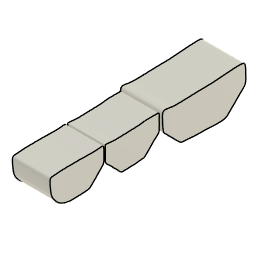
biomechanical finger (Autodesk Fusion 360 design; units mm, degrees)
Autodesk Fusion 360 part; units mm, degrees
sketch "Sketch1" plane through (0, 0, 0) normal (1, 0, 0) x (0, 1, 0)
  line L0 (-19, 9) -> (19, 9)
  line L1 (19, 9) -> (19, -9)
  line L2 (19, -9) -> (-19, -9)
  line L3 (-19, -9) -> (-19, 9)
  line L4 (-19, 9) -> (19, -9) construction
  line L5 (19, 9) -> (-19, -9) construction
  line L6 (-19, 0) -> (-44, 0) construction
  line L7 (-44, 0) -> (-69, 0) construction
  line L8 (-44, 0) -> (-44, 7.5)
  line L9 (-44, 7.5) -> (-19, 7.5)
  line L10 (-44, -7.5) -> (-19, -7.5)
  line L11 (-44, 0) -> (-44, -7.5)
  line L12 (-69, 0) -> (-69, 7.5)
  line L13 (-69, 7.5) -> (-44, 7.5)
  line L14 (-69, -7.5) -> (-44, -7.5)
  line L15 (-69, 0) -> (-69, -7.5)
  dimension "d1" = 38
  dimension "d2" = 18
  dimension "d3" = 25
  dimension "d4" = 25
  dimension "d5" = 7.5
  constraint horizontal L0
  constraint perpendicular L0 L1
  constraint parallel L0 L2
  constraint parallel L1 L3
  constraint coincident L4 origin
  constraint coincident L5 origin
  constraint midpoint L3 L6.start
  constraint perpendicular L3 L6
  constraint parallel L6 L7
  constraint perpendicular L7 L8
  constraint coincident L3 L9.end
  constraint perpendicular L3 L9
  constraint symmetric L7.start L6 L8.start
  constraint symmetric L6 L8.end L10.start
  constraint symmetric L6 L9.end L10.end
  constraint perpendicular L9 L12
  constraint perpendicular L8 L13
  constraint symmetric L12.start L7 L15.start
  constraint symmetric L7 L8.end L10.start
  constraint symmetric L7 L12.end L14.start
  measures "d1" distance of L0.start L0.end
  measures "d2" distance of L0.end L1.end
  measures "d3" distance of L6.start L6.end
  measures "d4" distance of L6.end L7.end
  measures "d5" distance of L6.end L8.end
sketch "Sketch2" plane through (0, 0, 0) normal (1, 0, 0) x (0, 1, 0)
  spline S0 degree 5 poles (26, 7) (25.7359, 7.0846) (25.2232, 7.2494) (24.5006, 7.4834) (23.6297, 7.7689) (22.6905, 8.0818) (21.884, 8.3509) (21.1781, 8.577) (20.5163, 8.7611) (19.8228, 8.9049) (19.0268, 9.0102) (18.0817, 9.0787) (16.9866, 9.1116) (15.7716, 9.1104) (14.4837, 9.0774) (13.1721, 9.0158) (11.8746, 8.9309) (10.602, 8.8299) (9.343, 8.7215) (8.0735, 8.6147) (6.764, 8.517) (5.3873, 8.4337) (3.9268, 8.3666) (2.3835, 8.3129) (0.7706, 8.267) (-0.8891, 8.2223) (-2.5676, 8.1727) (-4.2351, 8.1144) (-5.8638, 8.047) (-7.4316, 7.9759) (-8.9255, 7.9128) (-10.3394, 7.8724) (-11.6729, 7.8682) (-12.9294, 7.91) (-14.1153, 7.9996) (-15.2374, 8.1277) (-16.3028, 8.2707) (-17.3181, 8.3986) (-18.2905, 8.4817) (-19.228, 8.4975) (-20.1395, 8.4391) (-21.0354, 8.3162) (-21.9286, 8.1476) (-22.8349, 7.9564) (-23.7743, 7.7623) (-24.7697, 7.5788) (-25.8432, 7.4148) (-27.0111, 7.2746) (-28.2811, 7.159) (-29.6469, 7.0661) (-31.0894, 6.9921) (-32.5801, 6.9328) (-34.0848, 6.8844) (-35.5662, 6.8451) (-36.9876, 6.8158) (-38.3159, 6.802) (-39.5247, 6.8127) (-40.5987, 6.856) (-41.5367, 6.9349) (-42.3554, 7.0434) (-43.0947, 7.1607) (-43.8126, 7.254) (-44.5637, 7.2937) (-45.381, 7.2652) (-46.2562, 7.183) (-47.159, 7.0784) (-48.0575, 6.9862) (-48.9377, 6.9326) (-49.8227, 6.9228) (-50.7556, 6.9481) (-51.7839, 6.9924) (-52.9443, 7.038) (-54.2456, 7.0728) (-55.6718, 7.0903) (-57.1903, 7.0877) (-58.7578, 7.0655) (-60.3275, 7.0258) (-61.855, 6.9716) (-63.3064, 6.9054) (-64.6596, 6.8287) (-65.9014, 6.7425) (-66.8004, 6.6663) (-67.4206, 6.6051) (-67.8101, 6.5626) (-67.9988, 6.5409) knots 0 0 0 0 0 0 0.0125 0.025 0.0375 0.05 0.0625 0.075 0.0875 0.1 0.1125 0.125 0.1375 0.15 0.1625 0.175 0.1875 0.2 0.2125 0.225 0.2375 0.25 0.2625 0.275 0.2875 0.3 0.3125 0.325 0.3375 0.35 0.3625 0.375 0.3875 0.4 0.4125 0.425 0.4375 0.45 0.4625 0.475 0.4875 0.5 0.5125 0.525 0.5375 0.55 0.5625 0.575 0.5875 0.6 0.6125 0.625 0.6375 0.65 0.6625 0.675 0.6875 0.7 0.7125 0.725 0.7375 0.75 0.7625 0.775 0.7875 0.8 0.8125 0.825 0.8375 0.85 0.8625 0.875 0.8875 0.9 0.9125 0.925 0.9375 0.95 0.9625 0.975 0.9875 1 1 1 1 1 1
  spline S1 degree 5 poles (24.5129, -11.4787) (24.1663, -11.4324) (23.4806, -11.3421) (22.4736, -11.2136) (21.1745, -11.0562) (19.6223, -10.8825) (18.14, -10.7313) (16.7236, -10.6017) (15.3664, -10.492) (14.0584, -10.3994) (12.7852, -10.3205) (11.5285, -10.2504) (10.2679, -10.1839) (8.9836, -10.1157) (7.6581, -10.0412) (6.2784, -9.9568) (4.8385, -9.8605) (3.3396, -9.752) (1.7887, -9.6322) (0.1966, -9.5021) (-1.4231, -9.3632) (-3.0551, -9.2161) (-4.6844, -9.0606) (-6.2975, -8.8946) (-7.8824, -8.715) (-9.4273, -8.5182) (-10.9199, -8.3017) (-12.3462, -8.0641) (-13.6899, -7.807) (-14.9313, -7.5353) (-16.0458, -7.2582) (-17.0119, -6.9883) (-17.8199, -6.74) (-18.4796, -6.5277) (-19.0306, -6.365) (-19.544, -6.2627) (-20.1061, -6.2277) (-20.8056, -6.2621) (-21.7226, -6.3619) (-22.9187, -6.5182) (-24.4273, -6.7167) (-26.2439, -6.9382) (-28.3153, -7.1582) (-30.5528, -7.3503) (-32.846, -7.4887) (-35.0769, -7.551) (-37.1338, -7.5214) (-38.9249, -7.3935) (-40.3925, -7.1729) (-41.5257, -6.8802) (-42.3788, -6.555) (-43.0656, -6.2525) (-43.7166, -6.0257) (-44.4493, -5.9137) (-45.3253, -5.9238) (-46.3498, -6.0337) (-47.4939, -6.2059) (-48.71, -6.3983) (-49.9501, -6.5762) (-51.1823, -6.723) (-52.3873, -6.8359) (-53.5553, -6.9202) (-54.6829, -6.9853) (-55.7698, -7.0398) (-56.8154, -7.0861) (-57.8192, -7.1196) (-58.7823, -7.1298) (-59.7095, -7.1007) (-60.6106, -7.0114) (-61.5014, -6.8372) (-62.3961, -6.5559) (-63.3012, -6.153) (-64.2093, -5.6276) (-65.0915, -4.9979) (-65.9083, -4.2926) (-66.621, -3.54) (-67.2009, -2.76) (-67.643, -1.9517) (-67.9697, -1.0912) (-68.215, -0.1509) (-68.4131, 0.8859) (-68.5851, 2.0087) (-68.7257, 3.1629) (-68.8117, 4.2668) (-68.8115, 5.2302) (-68.6935, 5.9713) (-68.4881, 6.3444) (-68.2689, 6.4935) (-68.0937, 6.5348) (-67.9988, 6.5409) knots 0 0 0 0 0 0 0.01176471 0.02352941 0.03529412 0.04705882 0.05882353 0.07058824 0.08235294 0.09411765 0.10588235 0.11764706 0.12941176 0.14117647 0.15294118 0.16470588 0.17647059 0.18823529 0.2 0.21176471 0.22352941 0.23529412 0.24705882 0.25882353 0.27058824 0.28235294 0.29411765 0.30588235 0.31764706 0.32941176 0.34117647 0.35294118 0.36470588 0.37647059 0.38823529 0.4 0.41176471 0.42352941 0.43529412 0.44705882 0.45882353 0.47058824 0.48235294 0.49411765 0.50588235 0.51764706 0.52941176 0.54117647 0.55294118 0.56470588 0.57647059 0.58823529 0.6 0.61176471 0.62352941 0.63529412 0.64705882 0.65882353 0.67058824 0.68235294 0.69411765 0.70588235 0.71764706 0.72941176 0.74117647 0.75294118 0.76470588 0.77647059 0.78823529 0.8 0.81176471 0.82352941 0.83529412 0.84705882 0.85882353 0.87058824 0.88235294 0.89411765 0.90588235 0.91764706 0.92941176 0.94117647 0.95294118 0.96470588 0.97647059 0.98823529 1 1 1 1 1 1
  line L0 (-19, 0) -> (-8.3934, -10.6066)
  line L1 (-19, 0) -> (-4, 0) construction
  line L2 (-19, 0) -> (-29.6066, -10.6066)
  line L3 (-44, 0) -> (-33.3934, -10.6066)
  line L4 (-44, 0) -> (-29, 0) construction
  line L5 (-44, 0) -> (-54.6066, -10.6066)
  point P0 (21.4681, 8.4812)
  point P1 (19, 9)
  point P2 (13, 9)
  point P3 (5.5674, 8.4486)
  point P4 (-5.5989, 8.0568)
  point P5 (-14, 8)
  point P6 (-18.7896, 8.4812)
  point P7 (-22.4989, 8.0269)
  point P8 (-27.4654, 7.2378)
  point P9 (-36.4351, 6.8288)
  point P10 (-42, 7)
  point P11 (-44.602, 7.277)
  point P12 (-48, 7)
  point P13 (-52, 7)
  point P14 (-61, 7)
  point P15 (14.4554, -10.4292)
  point P16 (7, -10)
  point P17 (-3.6198, -9.1609)
  point P18 (-13.7888, -7.7778)
  point P19 (-18.2305, -6.6089)
  point P20 (-19.7695, -6.2583)
  point P21 (-24.5974, -6.7341)
  point P22 (-41, -7)
  point P23 (-44, -6)
  point P24 (-48.6731, -6.3884)
  point P25 (-55, -7)
  point P26 (-59.5398, -7.0955)
  point P27 (-63.3349, -6.1055)
  point P28 (-67, -3)
  point P29 (-68.4144, 0.9538)
  point P30 (-68.7145, 5.6867)
  dimension "d6" = 15
  dimension "d7" = 45
  dimension "d8" = 15
  dimension "d9" = 45
  dimension "d10" = 15
  dimension "d11" = 15
  constraint horizontal L1
  constraint perpendicular L0 L2
  constraint horizontal L4
  constraint perpendicular L3 L5
  measures "d6" distance of L0.start L0.end
  measures "d7" angle of L0 L1
  measures "d8" distance of L0.start L2.end
  measures "d9" angle of L3 L4
  measures "d10" distance of L3.start L3.end
  measures "d11" distance of L3.start L5.end
sketch "Sketch3" plane through (0, 0, 0) normal (1, 0, 0) x (0, 1, 0)
  line L0 (19, 0) -> (4.8579, -14.1421)
  line L1 (19, 0) -> (39, 0) construction
  spline S0 degree 5 poles (18.7905, 3.9439) (18.7865, 4.0757) (18.7799, 4.3324) (18.775, 4.6965) (18.7768, 5.1441) (18.7768, 5.6677) (18.7558, 6.1839) (18.7014, 6.7074) (18.617, 7.2245) (18.5082, 7.705) (18.371, 8.1156) (18.1733, 8.4349) (17.8568, 8.6602) (17.3674, 8.7995) (16.6863, 8.8672) (15.8406, 8.8791) (14.8845, 8.8522) (13.8863, 8.8026) (12.9137, 8.7442) (12.0208, 8.6872) (11.2309, 8.6367) (10.5315, 8.592) (9.8892, 8.5489) (9.2595, 8.5024) (8.5991, 8.4478) (7.8778, 8.3833) (7.0854, 8.3112) (6.2256, 8.2359) (5.3119, 8.1632) (4.3633, 8.0988) (3.3998, 8.047) (2.4381, 8.0097) (1.4884, 7.9854) (0.5564, 7.9708) (-0.3561, 7.9611) (-1.2498, 7.9515) (-2.1273, 7.9378) (-2.9915, 7.9172) (-3.8451, 7.8896) (-4.69, 7.8569) (-5.5276, 7.822) (-6.3586, 7.788) (-7.1833, 7.7578) (-8.0012, 7.7324) (-8.8114, 7.7111) (-9.613, 7.6918) (-10.405, 7.6728) (-11.1878, 7.6543) (-11.9626, 7.6398) (-12.7328, 7.6376) (-13.5035, 7.6611) (-14.2779, 7.7221) (-15.0552, 7.8257) (-15.8268, 7.9644) (-16.5744, 8.1127) (-17.2652, 8.22) (-17.8596, 8.2224) (-18.3234, 8.0626) (-18.6364, 7.7051) (-18.806, 7.1586) (-18.8647, 6.4717) (-18.8555, 5.711) (-18.8211, 4.9433) (-18.792, 4.2172) (-18.7736, 3.5433) (-18.7558, 2.9082) (-18.7226, 2.2914) (-18.6613, 1.6789) (-18.5743, 1.0823) (-18.4826, 0.5445) (-18.4048, 0.107) (-18.343, -0.2127) (-18.2594, -0.4566) (-18.0873, -0.7135) (-17.7736, -1.0621) (-17.3019, -1.5392) (-16.6829, -2.151) (-15.9472, -2.8786) (-15.1381, -3.6864) (-14.3041, -4.5291) (-13.4913, -5.3588) (-12.7365, -6.1323) (-12.0658, -6.813) (-11.4917, -7.3738) (-11.0115, -7.7993) (-10.605, -8.0882) (-10.2325, -8.2561) (-9.8325, -8.338) (-9.3436, -8.3753) (-8.7216, -8.406) (-7.9645, -8.4509) (-7.1067, -8.5138) (-6.2016, -8.5881) (-5.3075, -8.6613) (-4.472, -8.7205) (-3.7178, -8.7569) (-3.0258, -8.7717) (-2.3482, -8.7732) (-1.624, -8.7729) (-0.7943, -8.7826) (0.1834, -8.8108) (1.3181, -8.8589) (2.5811, -8.92) (3.9205, -8.9821) (5.2689, -9.0296) (6.5549, -9.0455) (7.7125, -9.013) (8.6919, -8.9182) (9.4684, -8.7517) (10.0552, -8.5109) (10.5042, -8.2005) (10.8846, -7.8294) (11.2654, -7.408) (11.6963, -6.9451) (12.1926, -6.446) (12.7469, -5.9143) (13.3372, -5.3543) (13.9368, -4.7721) (14.5226, -4.1778) (15.0856, -3.5876) (15.6268, -3.0197) (16.1516, -2.4898) (16.6645, -2.0058) (17.1644, -1.5645) (17.638, -1.1444) (18.0606, -0.709) (18.4058, -0.22) (18.6531, 0.3522) (18.7966, 1.0165) (18.8519, 1.7509) (18.8474, 2.5159) (18.8222, 3.1159) (18.8041, 3.5417) (18.7946, 3.8121) (18.7905, 3.9439) knots 0 0 0 0 0 0 0.00769231 0.01538462 0.02307692 0.03076923 0.03846154 0.04615385 0.05384615 0.06153846 0.06923077 0.07692308 0.08461538 0.09230769 0.1 0.10769231 0.11538462 0.12307692 0.13076923 0.13846154 0.14615385 0.15384615 0.16153846 0.16923077 0.17692308 0.18461538 0.19230769 0.2 0.20769231 0.21538462 0.22307692 0.23076923 0.23846154 0.24615385 0.25384615 0.26153846 0.26923077 0.27692308 0.28461538 0.29230769 0.3 0.30769231 0.31538462 0.32307692 0.33076923 0.33846154 0.34615385 0.35384615 0.36153846 0.36923077 0.37692308 0.38461538 0.39230769 0.4 0.40769231 0.41538462 0.42307692 0.43076923 0.43846154 0.44615385 0.45384615 0.46153846 0.46923077 0.47692308 0.48461538 0.49230769 0.5 0.50769231 0.51538462 0.52307692 0.53076923 0.53846154 0.54615385 0.55384615 0.56153846 0.56923077 0.57692308 0.58461538 0.59230769 0.6 0.60769231 0.61538462 0.62307692 0.63076923 0.63846154 0.64615385 0.65384615 0.66153846 0.66923077 0.67692308 0.68461538 0.69230769 0.7 0.70769231 0.71538462 0.72307692 0.73076923 0.73846154 0.74615385 0.75384615 0.76153846 0.76923077 0.77692308 0.78461538 0.79230769 0.8 0.80769231 0.81538462 0.82307692 0.83076923 0.83846154 0.84615385 0.85384615 0.86153846 0.86923077 0.87692308 0.88461538 0.89230769 0.9 0.90769231 0.91538462 0.92307692 0.93076923 0.93846154 0.94615385 0.95384615 0.96153846 0.96923077 0.97692308 0.98461538 0.99230769 1 1 1 1 1 1
  spline S1 degree 5 poles (-19.3, 4) (-19.2981, 3.9289) (-19.2948, 3.7885) (-19.2912, 3.5839) (-19.2897, 3.3237) (-19.2924, 3.0125) (-19.2974, 2.7044) (-19.3019, 2.3887) (-19.3038, 2.0604) (-19.3024, 1.7215) (-19.2988, 1.3786) (-19.2963, 1.0397) (-19.3014, 0.7124) (-19.3242, 0.4007) (-19.3771, 0.1047) (-19.4719, -0.1779) (-19.6169, -0.4502) (-19.8136, -0.7148) (-20.0552, -0.973) (-20.3295, -1.2253) (-20.622, -1.4722) (-20.9184, -1.7145) (-21.208, -1.954) (-21.4861, -2.1941) (-21.7522, -2.4388) (-22.009, -2.6917) (-22.2602, -2.9545) (-22.5096, -3.227) (-22.7591, -3.5049) (-23.009, -3.782) (-23.2586, -4.0517) (-23.507, -4.3093) (-23.7532, -4.553) (-23.9973, -4.7873) (-24.2399, -5.0205) (-24.482, -5.2615) (-24.7249, -5.5163) (-24.9694, -5.7845) (-25.2154, -6.0553) (-25.463, -6.3103) (-25.7121, -6.5295) (-25.964, -6.6966) (-26.2213, -6.8043) (-26.4893, -6.8604) (-26.7743, -6.8827) (-27.0828, -6.8929) (-27.4202, -6.9102) (-27.7895, -6.9445) (-28.1906, -6.9964) (-28.6213, -7.0604) (-29.0771, -7.1275) (-29.5515, -7.188) (-30.0363, -7.2344) (-30.5219, -7.264) (-30.9977, -7.279) (-31.4543, -7.2844) (-31.8843, -7.2866) (-32.284, -7.2917) (-32.654, -7.304) (-33.0018, -7.3243) (-33.3406, -7.3494) (-33.6845, -7.3743) (-34.0446, -7.3939) (-34.4251, -7.4048) (-34.8183, -7.4074) (-35.2038, -7.406) (-35.558, -7.4048) (-35.8612, -7.4047) (-36.1047, -7.4002) (-36.301, -7.3745) (-36.4827, -7.3014) (-36.6863, -7.1565) (-36.9391, -6.9266) (-37.2468, -6.6181) (-37.6004, -6.2503) (-37.9811, -5.8506) (-38.3651, -5.449) (-38.729, -5.0729) (-39.0548, -4.742) (-39.3357, -4.4623) (-39.5772, -4.2248) (-39.7924, -4.0127) (-39.9983, -3.8057) (-40.2119, -3.585) (-40.4458, -3.3397) (-40.7069, -3.0677) (-40.9973, -2.7724) (-41.3145, -2.4612) (-41.6518, -2.1425) (-41.9991, -1.8241) (-42.343, -1.51) (-42.6687, -1.2018) (-42.9618, -0.8997) (-43.2099, -0.6032) (-43.405, -0.313) (-43.5444, -0.0316) (-43.6335, 0.2354) (-43.6828, 0.4832) (-43.7046, 0.7116) (-43.7106, 0.9301) (-43.7086, 1.1607) (-43.7037, 1.4297) (-43.6987, 1.7593) (-43.6951, 2.1587) (-43.6934, 2.6174) (-43.6936, 3.1134) (-43.6953, 3.6179) (-43.6976, 4.1017) (-43.6999, 4.5408) (-43.7013, 4.9223) (-43.7017, 5.2508) (-43.7011, 5.543) (-43.7, 5.8179) (-43.6996, 6.0895) (-43.7017, 6.3564) (-43.7075, 6.5998) (-43.709, 6.7966) (-43.6833, 6.9297) (-43.5836, 7.0005) (-43.3618, 7.022) (-43.0011, 7.0076) (-42.5161, 6.9692) (-41.9411, 6.9172) (-41.3225, 6.8606) (-40.7095, 6.8064) (-40.1447, 6.76) (-39.6563, 6.7248) (-39.247, 6.7017) (-38.8975, 6.6902) (-38.5763, 6.6883) (-38.2475, 6.6934) (-37.8799, 6.7029) (-37.4555, 6.7148) (-36.9747, 6.7279) (-36.4496, 6.7417) (-35.9004, 6.7562) (-35.3505, 6.7716) (-34.8222, 6.788) (-34.3321, 6.8057) (-33.886, 6.8243) (-33.4772, 6.8433) (-33.0913, 6.8617) (-32.71, 6.8787) (-32.3154, 6.8938) (-31.8939, 6.9066) (-31.4409, 6.9178) (-30.9614, 6.9284) (-30.4667, 6.9398) (-29.9715, 6.9539) (-29.4913, 6.972) (-29.0393, 6.9955) (-28.6243, 7.025) (-28.2465, 7.0603) (-27.9005, 7.1007) (-27.5764, 7.1447) (-27.2626, 7.1908) (-26.9473, 7.2372) (-26.6214, 7.2822) (-26.2781, 7.3242) (-25.9126, 7.3617) (-25.5218, 7.3937) (-25.104, 7.4194) (-24.6583, 7.4384) (-24.1851, 7.4508) (-23.6865, 7.4569) (-23.167, 7.4579) (-22.6338, 7.4548) (-22.0975, 7.4496) (-21.5722, 7.4444) (-21.077, 7.4418) (-20.6324, 7.4437) (-20.2565, 7.4491) (-19.9613, 7.4526) (-19.7491, 7.4428) (-19.608, 7.3996) (-19.5114, 7.2963) (-19.4339, 7.1178) (-19.3674, 6.8802) (-19.316, 6.6187) (-19.2875, 6.3677) (-19.284, 6.1412) (-19.2971, 5.9232) (-19.3152, 5.6877) (-19.3275, 5.4107) (-19.3297, 5.0884) (-19.3227, 4.7322) (-19.3131, 4.4352) (-19.306, 4.215) (-19.3019, 4.0711) (-19.3, 4) knots 0 0 0 0 0 0 0.00540541 0.01081081 0.01621622 0.02162162 0.02702703 0.03243243 0.03783784 0.04324324 0.04864865 0.05405405 0.05945946 0.06486486 0.07027027 0.07567568 0.08108108 0.08648649 0.09189189 0.0972973 0.1027027 0.10810811 0.11351351 0.11891892 0.12432432 0.12972973 0.13513514 0.14054054 0.14594595 0.15135135 0.15675676 0.16216216 0.16756757 0.17297297 0.17837838 0.18378378 0.18918919 0.19459459 0.2 0.20540541 0.21081081 0.21621622 0.22162162 0.22702703 0.23243243 0.23783784 0.24324324 0.24864865 0.25405405 0.25945946 0.26486486 0.27027027 0.27567568 0.28108108 0.28648649 0.29189189 0.2972973 0.3027027 0.30810811 0.31351351 0.31891892 0.32432432 0.32972973 0.33513514 0.34054054 0.34594595 0.35135135 0.35675676 0.36216216 0.36756757 0.37297297 0.37837838 0.38378378 0.38918919 0.39459459 0.4 0.40540541 0.41081081 0.41621622 0.42162162 0.42702703 0.43243243 0.43783784 0.44324324 0.44864865 0.45405405 0.45945946 0.46486486 0.47027027 0.47567568 0.48108108 0.48648649 0.49189189 0.4972973 0.5027027 0.50810811 0.51351351 0.51891892 0.52432432 0.52972973 0.53513514 0.54054054 0.54594595 0.55135135 0.55675676 0.56216216 0.56756757 0.57297297 0.57837838 0.58378378 0.58918919 0.59459459 0.6 0.60540541 0.61081081 0.61621622 0.62162162 0.62702703 0.63243243 0.63783784 0.64324324 0.64864865 0.65405405 0.65945946 0.66486486 0.67027027 0.67567568 0.68108108 0.68648649 0.69189189 0.6972973 0.7027027 0.70810811 0.71351351 0.71891892 0.72432432 0.72972973 0.73513514 0.74054054 0.74594595 0.75135135 0.75675676 0.76216216 0.76756757 0.77297297 0.77837838 0.78378378 0.78918919 0.79459459 0.8 0.80540541 0.81081081 0.81621622 0.82162162 0.82702703 0.83243243 0.83783784 0.84324324 0.84864865 0.85405405 0.85945946 0.86486486 0.87027027 0.87567568 0.88108108 0.88648649 0.89189189 0.8972973 0.9027027 0.90810811 0.91351351 0.91891892 0.92432432 0.92972973 0.93513514 0.94054054 0.94594595 0.95135135 0.95675676 0.96216216 0.96756757 0.97297297 0.97837838 0.98378378 0.98918919 0.99459459 1 1 1 1 1 1
  spline S2 degree 5 poles (-44.3, 4) (-44.2999, 3.8618) (-44.2997, 3.5863) (-44.2988, 3.1792) (-44.2952, 2.6596) (-44.2878, 2.0645) (-44.2837, 1.5302) (-44.2942, 1.0544) (-44.3355, 0.6283) (-44.4287, 0.2377) (-44.5922, -0.1332) (-44.836, -0.4984) (-45.1524, -0.8654) (-45.5176, -1.2355) (-45.9032, -1.6073) (-46.2842, -1.9796) (-46.6499, -2.3549) (-47.0097, -2.7412) (-47.382, -3.1474) (-47.7852, -3.5798) (-48.2289, -4.0386) (-48.7024, -4.5126) (-49.176, -4.9805) (-49.6164, -5.4174) (-49.9975, -5.7996) (-50.3121, -6.11) (-50.5872, -6.3446) (-50.8805, -6.5125) (-51.2534, -6.6292) (-51.7499, -6.7116) (-52.3781, -6.7727) (-53.1219, -6.8225) (-53.9488, -6.8678) (-54.8185, -6.9124) (-55.6909, -6.9567) (-56.5359, -6.9984) (-57.3389, -7.032) (-58.0963, -7.0507) (-58.8124, -7.0469) (-59.4954, -7.014) (-60.1541, -6.947) (-60.7945, -6.8438) (-61.4159, -6.7066) (-62.0142, -6.5396) (-62.5838, -6.347) (-63.1209, -6.1315) (-63.6252, -5.892) (-64.1031, -5.622) (-64.5648, -5.3118) (-65.0203, -4.9524) (-65.4765, -4.5378) (-65.9333, -4.0692) (-66.3809, -3.5564) (-66.8046, -3.0139) (-67.1879, -2.4564) (-67.5167, -1.8948) (-67.7826, -1.3323) (-67.988, -0.7588) (-68.1441, -0.155) (-68.2664, 0.5004) (-68.3703, 1.2231) (-68.4674, 2.0165) (-68.5606, 2.864) (-68.641, 3.7231) (-68.6915, 4.537) (-68.6918, 5.2471) (-68.6224, 5.805) (-68.4686, 6.1839) (-68.2257, 6.3927) (-67.9011, 6.4807) (-67.5069, 6.5101) (-67.0538, 6.532) (-66.5464, 6.5679) (-65.9859, 6.6217) (-65.3722, 6.6853) (-64.7055, 6.7469) (-63.9885, 6.7987) (-63.2264, 6.8379) (-62.426, 6.8648) (-61.5947, 6.8822) (-60.74, 6.8935) (-59.8688, 6.9025) (-58.9865, 6.9112) (-58.0964, 6.9197) (-57.2007, 6.9268) (-56.3005, 6.9304) (-55.3967, 6.9285) (-54.4903, 6.9195) (-53.5829, 6.9032) (-52.6772, 6.881) (-51.7777, 6.8568) (-50.8903, 6.8363) (-50.0223, 6.8252) (-49.1823, 6.829) (-48.3801, 6.8514) (-47.626, 6.8931) (-46.9315, 6.9512) (-46.3087, 7.0178) (-45.7684, 7.0795) (-45.3187, 7.1172) (-44.9634, 7.106) (-44.6993, 7.0135) (-44.5166, 6.8042) (-44.401, 6.4543) (-44.3368, 5.9668) (-44.308, 5.368) (-44.3016, 4.831) (-44.3004, 4.4156) (-44.3001, 4.1382) (-44.3, 4) knots 0 0 0 0 0 0 0.00952381 0.01904762 0.02857143 0.03809524 0.04761905 0.05714286 0.06666667 0.07619048 0.08571429 0.0952381 0.1047619 0.11428571 0.12380952 0.13333333 0.14285714 0.15238095 0.16190476 0.17142857 0.18095238 0.19047619 0.2 0.20952381 0.21904762 0.22857143 0.23809524 0.24761905 0.25714286 0.26666667 0.27619048 0.28571429 0.2952381 0.3047619 0.31428571 0.32380952 0.33333333 0.34285714 0.35238095 0.36190476 0.37142857 0.38095238 0.39047619 0.4 0.40952381 0.41904762 0.42857143 0.43809524 0.44761905 0.45714286 0.46666667 0.47619048 0.48571429 0.4952381 0.5047619 0.51428571 0.52380952 0.53333333 0.54285714 0.55238095 0.56190476 0.57142857 0.58095238 0.59047619 0.6 0.60952381 0.61904762 0.62857143 0.63809524 0.64761905 0.65714286 0.66666667 0.67619048 0.68571429 0.6952381 0.7047619 0.71428571 0.72380952 0.73333333 0.74285714 0.75238095 0.76190476 0.77142857 0.78095238 0.79047619 0.8 0.80952381 0.81904762 0.82857143 0.83809524 0.84761905 0.85714286 0.86666667 0.87619048 0.88571429 0.8952381 0.9047619 0.91428571 0.92380952 0.93333333 0.94285714 0.95238095 0.96190476 0.97142857 0.98095238 0.99047619 1 1 1 1 1 1
  point P0 (18.7462, 6.2045)
  point P1 (18.4137, 7.9554)
  point P2 (17.5494, 8.7311)
  point P3 (12.3633, 8.7089)
  point P4 (8.8173, 8.4651)
  point P5 (3.7199, 8.0662)
  point P6 (-2.264, 7.9332)
  point P7 (-7.2728, 7.7559)
  point P8 (-11.7718, 7.6451)
  point P9 (-16, 8)
  point P10 (-18.4378, 7.8855)
  point P11 (-18.8207, 4.9155)
  point P12 (-18.6734, 1.8418)
  point P13 (-18.3779, -0.0197)
  point P14 (-18.1029, -0.6706)
  point P15 (-14.4107, -4.423)
  point P16 (-10.6303, -8.0481)
  point P17 (-9.1285, -8.3847)
  point P18 (-4.4172, -8.7192)
  point P19 (-0.2694, -8.7996)
  point P20 (9.1719, -8.7996)
  point P21 (11.2109, -7.4699)
  point P22 (14.0034, -4.6995)
  point P23 (16.9288, -1.774)
  point P24 (18.6132, 0.3314)
  point P25 (-19.3, 2.5)
  point P26 (-19.3, 0.9)
  point P27 (-19.6, -0.4)
  point P28 (-20.9, -1.7)
  point P29 (-22.3, -3)
  point P30 (-23.6, -4.4)
  point P31 (-24.8, -5.6)
  point P32 (-26, -6.7)
  point P33 (-27.2, -6.9)
  point P34 (-29.7, -7.2)
  point P35 (-32.5, -7.3)
  point P36 (-34.3, -7.4)
  point P37 (-36, -7.4)
  point P38 (-36.6641, -7.1629)
  point P39 (-38.9, -4.9)
  point P40 (-40.1, -3.7)
  point P41 (-41.7, -2.1)
  point P42 (-43.4, -0.3)
  point P43 (-43.7, 0.7)
  point P44 (-43.7, 1.7)
  point P45 (-43.7, 4.6)
  point P46 (-43.7, 6)
  point P47 (-43.7, 6.8)
  point P48 (-43.5, 7)
  point P49 (-40.001, 6.7505)
  point P50 (-38, 6.7)
  point P51 (-34.5, 6.8)
  point P52 (-32.1, 6.9)
  point P53 (-29, 7)
  point P54 (-27.2, 7.2)
  point P55 (-25.4, 7.4)
  point P56 (-21.9918, 7.4486)
  point P57 (-19.8092, 7.44)
  point P58 (-19.5, 7.25)
  point P59 (-19.3, 6.45)
  point P60 (-19.3161, 5.6361)
  point P61 (-44.3, 1.1)
  point P62 (-44.7246, -0.317)
  point P63 (-46.2, -1.9)
  point P64 (-48, -3.8)
  point P65 (-50.1538, -5.9509)
  point P66 (-51.2, -6.6)
  point P67 (-55.4822, -6.9459)
  point P68 (-60.12, -6.9418)
  point P69 (-63.1543, -6.1072)
  point P70 (-65.4122, -4.5861)
  point P71 (-67.6, -1.7)
  point P72 (-68.4623, 1.9954)
  point P73 (-68.4902, 6.0683)
  point P74 (-67.6, 6.5)
  point P75 (-65.2, 6.7)
  point P76 (-60.1, 6.9)
  point P77 (-53.5, 6.9)
  point P78 (-47.6, 6.9)
  point P79 (-45.1, 7.1)
  point P80 (-44.5, 6.7)
  dimension "d12" = 135
  dimension "d13" = 20
  constraint horizontal L1
  measures "d12" angle of L0 L1
  measures "d13" distance of L0.start L0.end
extrude "Extrude1" add sketch "Sketch3" along normal mid plane 19 contours S0 makes body 1
extrude "Extrude2" add sketch "Sketch3" along normal mid plane 17 separate body contours S1 | S2 makes body 2 at (2.9383, -22.2685, -2.9663) makes body 3 at (5.8486, -46.4083, -2.1095)
